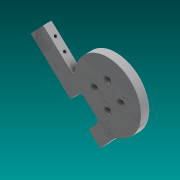
# Autodesk Inventor part: gearboxframv2
Saved by Autodesk Inventor 2020.2 (Build 242310000, 310)
## iProperties
Created: 2020-05-20
Part Number: gearboxframv2
Material: Aluminum 6061
Document SubType Name: Modeling
Designer: Svend
Density: 2.7 g/cm^3
Appearance: Aluminum - Polished
Author: Svend
Autodesk Inventor part; units mm, degrees
ref_plane "YZ Plane" through (0, 0, 0) normal (1, 0, 0) x (0, 1, 0)
ref_plane "XZ Plane" through (0, 0, 0) normal (0, 1, 0) x (-1, 0, 0)
ref_plane "XY Plane" through (0, 0, 0) normal (0, 0, 1) x (1, 0, 0)
ref_plane "Work Plane1" through (0, 0, 0) normal (0, 0, 1) x (1, 0, 0)
sketch "Sketch1" plane through (0, 0, 0) normal (0, 0, 1) x (1, 0, 0)
  arc A0 (-77.068, 33.987) -> (-78.4814, 33.9394) centre (-77.7509, 33.2565) ccw projected
  line L0 (-78.4814, 33.9394) -> (-92.9244, 18.4887) projected
  line L1 (-92.9244, 18.4887) -> (-45.0314, -26.2807) projected
  line L2 (-45.0314, -26.2807) -> (-35.471, -16.0534) projected
  arc A1 (-28.404, -15.8151) -> (-35.471, -16.0534) centre (-31.8184, -19.4678) ccw projected
  line L3 (-28.404, -15.8151) -> (-13.8665, -29.4045) projected
  arc A2 (-13.6283, -36.4716) -> (-13.8665, -29.4045) centre (-17.2809, -33.0572) ccw projected
  line L4 (-13.6283, -36.4716) -> (-23.1886, -46.699) projected
  line L5 (-23.1886, -46.699) -> (-9.2531, -59.7257) projected
  line L6 (-9.2531, -59.7257) -> (9.7389, -39.4086) projected
  arc A3 (10.6702, -38.8458) -> (9.7389, -39.4086) centre (11.2, -40.7744) ccw projected
  arc A4 (10.6702, -38.8458) -> (15.1663, -37.3207) centre (0, 0) ccw projected
  line L7 (15.1663, -37.3207) -> (23.5338, -32.6958) projected
  arc A5 (23.5338, -32.6958) -> (34.2063, -21.2786) centre (0, 0) ccw projected
  line L8 (34.2063, -21.2786) -> (38.2573, -12.6186) projected
  arc A6 (38.2573, -12.6186) -> (40.1807, 2.8912) centre (0, 0) ccw projected
  line L9 (40.1807, 2.8912) -> (38.3679, 12.2784) projected
  arc A7 (38.3679, 12.2784) -> (30.8075, 25.9567) centre (0, 0) ccw projected
  line L10 (30.8075, 25.9567) -> (23.8232, 32.4855) projected
  arc A8 (23.8232, 32.4855) -> (9.6668, 39.1076) centre (0, 0) ccw projected
  line L11 (9.6668, 39.1076) -> (0.1789, 40.2842) projected
  arc A9 (0.1789, 40.2842) -> (-15.1663, 37.3207) centre (0, 0) ccw projected
  line L12 (-15.1663, 37.3207) -> (-23.5338, 32.6958) projected
  arc A10 (-23.5338, 32.6958) -> (-34.2063, 21.2786) centre (0, 0) ccw projected
  line L13 (-34.2063, 21.2786) -> (-38.2573, 12.6186) projected
  arc A11 (-38.2573, 12.6186) -> (-40.1013, 3.8394) centre (0, 0) ccw projected
  arc A12 (-43.4579, 2.5689) -> (-40.1013, 3.8394) centre (-42.0921, 4.03) ccw projected
  line L14 (-43.4579, 2.5689) -> (-77.068, 33.987) projected
  circle A13 centre (33.3141, 1.123) radius 2.5 projected
  circle A14 centre (1.123, -33.3141) radius 2.5 projected
  circle A15 centre (0, 0) radius 21 projected
  circle A16 centre (-1.123, 33.3141) radius 2.5 projected
  circle A17 centre (-33.3141, -1.123) radius 2.5 projected
  circle A18 centre (0, 0) radius 12.5 projected
  circle A19 centre (0, -16) radius 2 projected
  circle A20 centre (0, 16) radius 2 projected
  circle A21 centre (-16, 0) radius 2 projected
  circle A22 centre (16, 0) radius 2 projected
  circle A23 centre (11.3137, 11.3137) radius 1.6 projected
  circle A24 centre (-11.3137, -11.3137) radius 1.6 projected
  circle A25 centre (-11.3137, 11.3137) radius 1.6 projected
  circle A26 centre (11.3137, -11.3137) radius 1.6 projected
  circle A27 centre (0, 0) radius 20.7 projected
  circle A28 centre (0, 0) radius 40.2846
  point P0 (0, 0)
  point P1 (-38.2573, 12.6186)
  point P2 (-34.2063, 21.2786)
  point P3 (-23.5338, 32.6958)
  point P4 (-15.1663, 37.3207)
  point P5 (-36.4666, -17.1184)
  point P6 (-14.6238, -37.5366)
  point P7 (23.5338, -32.6958)
  point P8 (15.1663, -37.3207)
  point P9 (38.2573, -12.6186)
  point P10 (34.2063, -21.2786)
  point P11 (40.1807, 2.8912)
  point P12 (23.8232, 32.4855)
  point P13 (30.8075, 25.9567)
  point P14 (9.6668, 39.1076)
  constraints: 1 centre point, 1 coincident
extrude "Extrusion1" add sketch "Sketch1" along normal blind 10 contours L14 A12 A28 L2 L1 L0 A0 | A11 L13 A10 L12 A9 L11 A8 L10 A7 L9 A6 L8 A5 L7 A4 A28 L4 A2 L3 A1 L2 | A28 L13 | A28 A3 L6 L5 L4 | A28 L12 | L7 A28 | A28 L11 | L8 A28 | A28 L10 | A28 L9 | A13 | A14 | A15 | A16 | A17 | A19 | A20 | A21 | A22 | A23 | A24 | A25 | A26 | A27
sketch "Sketch2" plane through (-77.068, 33.987, 10) normal (0.6828833, 0.7305275, 0) x (0.7305275, -0.6828833, 0)
  arc A0 (41, 70.5) -> (39, 72.5) centre (39, 70.5) ccw projected
  line L0 (1, 72.5) -> (39, 72.5) projected
  arc A1 (1, 72.5) -> (-1, 70.5) centre (1, 70.5) ccw projected
  line L1 (-1, 2) -> (-1, 70.5) projected
  arc A2 (-1, 2) -> (1, 0) centre (1, 2) ccw projected
  line L2 (39, 0) -> (1, 0) projected
  arc A3 (39, 0) -> (41, 2) centre (39, 2) ccw projected
  line L3 (41, 70.5) -> (41, 2) projected
  circle A4 centre (20, 36.25) radius 12.6 projected
  circle A5 centre (36, 36.25) radius 2 projected
  arc A6 (35.4, 2.9) -> (35.4, 7.1) centre (35.4, 5) ccw projected
  line L4 (4.6, 2.9) -> (35.4, 2.9) projected
  arc A7 (4.6, 7.1) -> (4.6, 2.9) centre (4.6, 5) ccw projected
  line L5 (35.4, 7.1) -> (4.6, 7.1) projected
  circle A8 centre (20, 20.25) radius 2 projected
  circle A9 centre (31.3137, 24.9363) radius 1.5 projected
  circle A10 centre (8.6863, 24.9363) radius 1.5 projected
  circle A11 centre (31.3137, 47.5637) radius 1.5 projected
  arc A12 (4.6, 69.6) -> (4.6, 65.4) centre (4.6, 67.5) ccw projected
  line L6 (35.4, 69.6) -> (4.6, 69.6) projected
  arc A13 (35.4, 65.4) -> (35.4, 69.6) centre (35.4, 67.5) ccw projected
  line L7 (4.6, 65.4) -> (35.4, 65.4) projected
  circle A14 centre (20, 52.25) radius 2 projected
  circle A15 centre (8.6863, 47.5637) radius 1.5 projected
  circle A16 centre (4, 36.25) radius 2 projected
  point P0 (79.5095, 10)
  point P1 (12.3, 5)
  point P2 (27.7, 5)
  dimension "d2" = 7.7
  dimension "d3" = 7.7
  constraints: 2 horizontal alignment
  measures "d2" distance of A7.centre point (12.3, 5)
  measures "d3" distance of point (27.7, 5) A6.centre
hole "Hole1" at (-68.0825, 25.5876, 5) at (-56.8324, 15.0712, 5) direction (-0.6828833, -0.7305275, 0) diameter 3.242 depth 22.15 tip angle 118 thread size "M4x0.7" class "6H" standard "ISO Metric profile"
sketch "Sketch3" plane through (0, 0, 10) normal (0, 0, 1) x (1, 0, 0)
  circle A0 centre (0, 0) radius 12.5 projected
  circle A1 centre (0, -16) radius 2 projected
  circle A2 centre (0, 16) radius 2 projected
  circle A3 centre (-16, 0) radius 2 projected
  circle A4 centre (16, 0) radius 2 projected
  circle A5 centre (11.3137, 11.3137) radius 1.6 projected
  circle A6 centre (-11.3137, -11.3137) radius 1.6 projected
  circle A7 centre (-11.3137, 11.3137) radius 1.6 projected
  circle A8 centre (11.3137, -11.3137) radius 1.6 projected
  circle A9 centre (0, 0) radius 20.7 projected
  point P0 (0, 0)
hole "Hole2" at (0, 16, 10) at (16, 0, 10) at (0, -16, 10) at (-16, 0, 10) direction (0, 0, -1) diameter 4.5 end through all countersink diameter 8.5 countersink angle 90 clearance for "Countersunk Flat Head Screw ISO 2009/7046" size "M4" standard "ISO"
sketch "Sketch4" plane through (-45.0314, -26.2807, 0) normal (-0.6828833, -0.7305275, 0) x (0.7305275, -0.6828833, 0)
  circle A0 centre (-11.576, 5) radius 2.067 projected
  circle A1 centre (41.476, 5) radius 2.067 projected
  point P0 (14.95, 0)
hole "Hole3" at (-53.488, -18.3757, 5) at (-14.732, -54.604, 5) direction (0.6828833, 0.7305275, 0) diameter 3.242 depth 19 tip angle 118 thread size "M4x0.7" class "6H" standard "ISO Metric profile"
equation "\"d3\" = d2"
body "Solid1"
